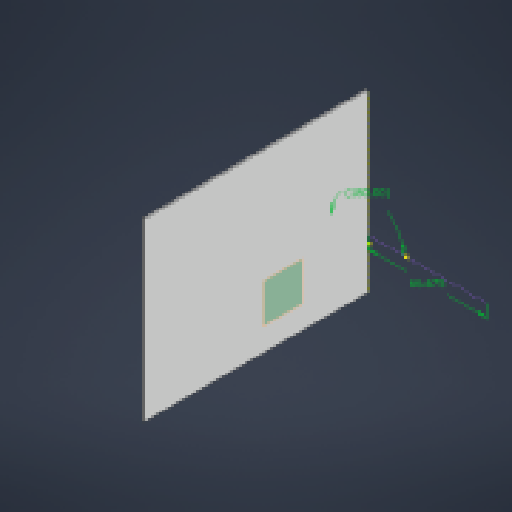
# Autodesk Inventor part: the wall
Saved by Autodesk Inventor 2025 (Build 290162000, 162)
## iProperties
Created: 2024-08-17
Part Number: the wall
Material: Generic
Document SubType Name: Modeling
Designer: Windows 7 was better
Density: 1 g/cm^3
Appearance: Default
Author: Windows 7 was better
Autodesk Inventor part; units mm, degrees
ref_plane "YZ Plane" through (0, 0, 0) normal (1, 0, 0) x (0, 1, 0)
ref_plane "XZ Plane" through (0, 0, 0) normal (0, 1, 0) x (-1, 0, 0)
ref_plane "XY Plane" through (0, 0, 0) normal (0, 0, 1) x (1, 0, 0)
ref_plane "Work Plane1" through (-0.4619, 0, 36.47) normal (-1, 0, 0) x (0, 0, 1)
sketch "Sketch2" plane through (-0.4619, 0, 36.47) normal (-1, 0, 0) x (0, 0, 1)
  line L0 (77.2498, 74.2499) -> (-47.6281, 74.2499)
  line L1 (-47.6281, 74.2499) -> (-47.6281, -23.9656)
  line L2 (-47.6281, -23.9656) -> (77.2498, -23.9656)
  line L3 (77.2498, -23.9656) -> (77.2498, 74.2499)
  point P0 (-36.47, 0)
  constraints: 8 end point, 2 parallel, 1 horizontal, 1 perpendicular
extrude "Extrusion2" add sketch "Sketch2" along normal blind 1
sketch "Sketch4" plane through (-0.4619, -23.9656, -11.1581) normal (0, 0, -1) x (-1, 0, 0)
  line L0 (0, 98.2155) -> (0, 0) projected
  line L1 (0, 28.2273) -> (-66.675, 28.2273)
  line L2 (0, 28.2273) -> (66.675, 28.2273) construction
  point P0 (-0.4619, 23.9656)
  dimension "d8" = 66.675
  dimension "d9" = 180
  constraints: 4 end point, 1 collinear, 1 horizontal, 1 perpendicular, 1 point on line
  measures "d8" distance of L1.start L1.end
  measures "d9" angle of L1 L2
body "Solid1"
